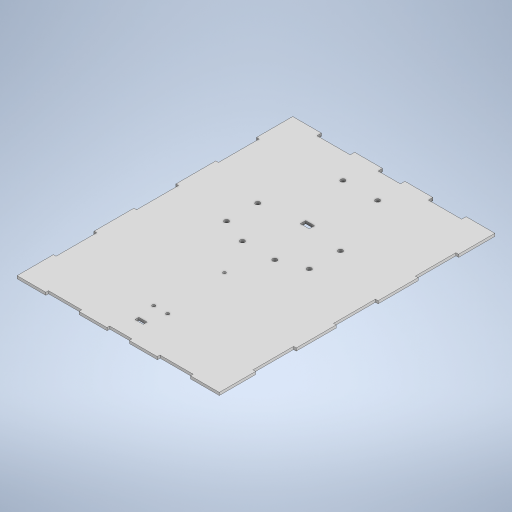
# Autodesk Inventor part: totalPart
Saved by Autodesk Inventor 2023 (Build 270158000, 158)
## iProperties
Created: 2022-11-20
Part Number: totalPart
Material: Generic
Document SubType Name: Modeling
Designer: ADMIN
Density: 1 g/cm^3
Appearance: Default
Author: ADMIN
Autodesk Inventor part; units mm, degrees
ref_plane "YZ Plane" through (0, 0, 0) normal (1, 0, 0) x (0, 1, 0)
ref_plane "XZ Plane" through (0, 0, 0) normal (0, 1, 0) x (-1, 0, 0)
ref_plane "XY Plane" through (0, 0, 0) normal (0, 0, 1) x (1, 0, 0)
sketch "Sketch1" plane through (0, 0, 0) normal (0, 1, 0) x (-1, 0, 0)
  line L0 (48.8824, 24.5697) -> (45.8824, 24.5697)
  line L1 (48.8824, -65.4156) -> (45.8824, -65.4156)
  line L2 (48.8824, -20.7764) -> (45.8824, -20.7764)
  line L3 (48.8824, -202.2369) -> (45.8824, -202.2369)
  line L4 (48.8824, -112.2516) -> (45.8824, -112.2516)
  line L5 (48.8824, -156.8908) -> (45.8824, -156.8908)
  line L6 (48.8824, 24.5697) -> (48.8824, 62.1664)
  line L7 (48.8824, 24.5697) -> (48.8824, 65.1664)
  line L8 (48.8824, -65.4156) -> (48.8824, -20.7764)
  line L9 (48.8824, -65.4156) -> (48.8824, -20.7764)
  line L10 (48.8824, -237.8336) -> (48.8824, -202.2369)
  line L11 (48.8824, -156.8908) -> (48.8824, -112.2516)
  line L12 (48.8824, -242.8336) -> (48.8824, -202.2369)
  line L13 (48.8824, -156.8908) -> (48.8824, -112.2516)
  line L14 (45.8824, -20.7764) -> (45.8824, 24.5697)
  line L15 (45.8824, -202.2369) -> (45.8824, -156.8908)
  line L16 (45.8824, -112.2516) -> (45.8824, -65.4156)
  line L17 (-177.1176, 24.5697) -> (-174.1176, 24.5697)
  line L18 (-177.1176, -65.4156) -> (-174.1176, -65.4156)
  line L19 (-177.1176, -20.7764) -> (-174.1176, -20.7764)
  line L20 (-177.1176, -202.2369) -> (-174.1176, -202.2369)
  line L21 (-177.1176, -156.8908) -> (-174.1176, -156.8908)
  line L22 (-177.1176, -112.2516) -> (-174.1176, -112.2516)
  line L23 (-177.1176, 65.1664) -> (-177.1176, 24.5697)
  line L24 (-174.1176, 24.5697) -> (-174.1176, -20.7764)
  line L25 (-177.1176, -20.7764) -> (-177.1176, -65.4156)
  line L26 (-174.1176, -65.4156) -> (-174.1176, -112.2516)
  line L27 (-174.1176, -156.8908) -> (-174.1176, -202.2369)
  line L28 (-177.1176, -112.2516) -> (-177.1176, -156.8908)
  line L29 (-177.1176, -202.2369) -> (-177.1176, -242.8336)
  line L30 (48.8824, -237.8336) -> (48.8824, -242.8336)
  line L31 (16.7044, 65.1664) -> (16.7044, 62.1664)
  line L32 (-20.3174, 65.1664) -> (-20.3174, 62.1664)
  line L33 (-51.677, 65.1664) -> (-51.677, 62.1664)
  line L34 (-144.9395, 65.1664) -> (-144.9395, 62.1664)
  line L35 (-107.9177, 65.1664) -> (-107.9177, 62.1664)
  line L36 (-76.5581, 65.1664) -> (-76.5581, 62.1664)
  line L37 (48.8824, 65.1664) -> (16.7044, 65.1664)
  line L38 (-64.1176, 62.1664) -> (-51.677, 62.1664)
  line L39 (-20.3174, 62.1664) -> (16.7044, 62.1664)
  line L40 (16.7044, 62.1664) -> (-20.3174, 62.1664)
  line L41 (-20.3174, 65.1664) -> (-51.677, 65.1664)
  line L42 (-51.677, 62.1664) -> (-76.5581, 62.1664)
  line L43 (-107.9177, 62.1664) -> (-144.9395, 62.1664)
  line L44 (-64.1176, 62.1664) -> (-76.5581, 62.1664)
  line L45 (-76.5581, 65.1664) -> (-107.9177, 65.1664)
  line L46 (-144.9395, 65.1664) -> (-177.1176, 65.1664)
  line L47 (16.7044, -242.8336) -> (16.7044, -237.8336)
  line L48 (-20.3174, -242.8336) -> (-20.3174, -237.8336)
  line L49 (-51.677, -242.8336) -> (-51.677, -237.8336)
  line L50 (-144.9395, -242.8336) -> (-144.9395, -237.8336)
  line L51 (-107.9177, -242.8336) -> (-107.9177, -237.8336)
  line L52 (-76.5581, -242.8336) -> (-76.5581, -237.8336)
  line L53 (-177.1176, -242.8336) -> (-144.9395, -242.8336)
  line L54 (-144.9395, -237.8336) -> (-107.9177, -237.8336)
  line L55 (-107.9177, -242.8336) -> (-76.5581, -242.8336)
  line L56 (-76.5581, -237.8336) -> (-51.677, -237.8336)
  line L57 (-51.677, -242.8336) -> (-20.3174, -242.8336)
  line L58 (16.7044, -242.8336) -> (48.8824, -242.8336)
  line L59 (-20.3174, -237.8336) -> (16.7044, -237.8336)
  line L60 (-64.1176, 62.1664) -> (-64.1176, 17.1664)
  line L61 (-64.1176, 17.1664) -> (-64.1176, 17.9164)
  line L62 (-64.1176, 17.9164) -> (-56.6176, 17.9164)
  circle A0 centre (-56.6176, 17.9164) radius 1.75
  circle A1 centre (-72.1176, 17.9164) radius 1.75
  line L63 (-68.6972, 41.8347) -> (-59.538, 41.8347)
  line L64 (-59.538, 41.8347) -> (-59.538, 37.4981)
  line L65 (-59.538, 37.4981) -> (-68.6972, 37.4981)
  line L66 (-68.6972, 37.4981) -> (-68.6972, 41.8347)
  line L67 (-68.6972, 41.8347) -> (-59.538, 37.4981) construction
  line L68 (-59.538, 41.8347) -> (-68.6972, 37.4981) construction
  circle A2 centre (-64.1176, -53.5615) radius 1.6
  line L69 (-69.1176, -149.3399) -> (-59.1176, -149.3399)
  line L70 (-59.1176, -149.3399) -> (-59.1176, -143.3399)
  line L71 (-59.1176, -143.3399) -> (-69.1176, -143.3399)
  line L72 (-69.1176, -143.3399) -> (-69.1176, -149.3399)
  line L73 (-69.1176, -149.3399) -> (-59.1176, -143.3399) construction
  line L74 (-59.1176, -149.3399) -> (-69.1176, -143.3399) construction
  circle A3 centre (-107.9177, -104.5303) radius 2.5
  circle A4 centre (-107.9177, -139.4281) radius 2.5
  circle A5 centre (-15.5025, -104.5303) radius 2.5
  circle A6 centre (-15.5025, -139.4281) radius 2.5
  circle A7 centre (-79.8847, -94.0776) radius 2.5
  circle A8 centre (-43.6456, -94.0776) radius 2.5
  circle A9 centre (-79.8847, -208.9633) radius 2.5
  circle A10 centre (-41.1456, -208.9633) radius 2.5
  point P0 (0, 0)
  point P1 (-20.3174, -239.8336)
  point P2 (-51.677, -239.8336)
  point P3 (-107.9177, -239.8336)
  point P4 (-76.5581, -239.8336)
  point P5 (16.7044, -239.8336)
  point P6 (-144.9395, -239.8336)
  point P7 (-126.4286, -237.8336)
  point P8 (-126.4286, 62.1664)
  point P9 (-161.0285, 65.1664)
  point P10 (-174.1176, -179.5638)
  point P11 (-64.1176, 39.6664)
  point P12 (-64.1176, -146.3399)
  dimension "d0" = 226
  dimension "d1" = 308
  dimension "d11" = 300
  dimension "d15" = 220
  dimension "d16" = 5
  dimension "d19" = 45
  dimension "d20" = 0.75
  dimension "d21" = 7.5
  dimension "d22" = 3.5
  dimension "d23" = 3.5
  dimension "d24" = 15.5
  dimension "d25" = 3.2
  dimension "d26" = 10
  dimension "d27" = 6
  dimension "d28" = 5
  dimension "d29" = 5
  dimension "d30" = 5
  dimension "d31" = 5
  dimension "d32" = 5
  dimension "d33" = 5
  dimension "d34" = 5
  dimension "d35" = 5
  constraints: 150 end point, 48 parallel, 40 perpendicular, 12 horizontal, 11 centre point, 9 midpoint, 8 point on line, 1 coincident, 1 collinear, 1 vertical
  measures "d0" distance of L12.start L29.end
  measures "d1" distance of L29.end L23.start
  measures "d11" distance of point (-126.429, -237.834) point (-126.429, 62.166)
  measures "d15" distance from line of point (-174.118, -179.564) L15
  measures "d16" distance of L47.start L47.end
  measures "d19" distance of L38.start L60.end
  measures "d20" distance of L60.end L61.end
  measures "d21" distance of L61.end L62.end
  measures "d22" diameter of A0
  measures "d23" diameter of A1
  measures "d24" distance of A1.centre L62.end
  measures "d25" diameter of A2
  measures "d26" distance of L71.end L70.end
  measures "d27" distance of L70.end L69.end
  measures "d28" diameter of A3
  measures "d29" diameter of A4
  measures "d30" diameter of A5
  measures "d31" diameter of A6
  measures "d32" diameter of A7
  measures "d33" diameter of A8
  measures "d34" diameter of A9
  measures "d35" diameter of A10
extrude "Extrusion1" add sketch "Sketch1" along normal blind 3
body "Solid1"
